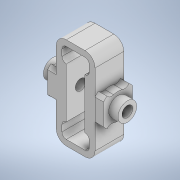
# Autodesk Inventor part: Součást3
Saved by Autodesk Inventor 2022 (Build 260153000, 153)
## iProperties
Created: 2022-04-03
Part Number: Součást3
Material: Všeobecné
Document SubType Name: Modeling
Designer: Šimon
Density: 1 g/cm^3
Appearance: Výchozí
Author: Šimon
Autodesk Inventor part; units mm, degrees
ref_plane "YZ Plane" through (0, 0, 0) normal (1, 0, 0) x (0, 1, 0)
ref_plane "XZ Plane" through (0, 0, 0) normal (0, 1, 0) x (-1, 0, 0)
ref_plane "XY Plane" through (0, 0, 0) normal (0, 0, 1) x (1, 0, 0)
sketch "Náčrt2" plane through (0, 0, 0) normal (0, 0, 1) x (1, 0, 0)
  line L0 (0, 0) -> (54, 0)
  line L1 (54, 0) -> (54, 128)
  line L2 (54, 128) -> (0, 128)
  line L3 (0, 128) -> (0, 0)
  line L4 (8, 120) -> (46, 120)
  line L5 (46, 120) -> (46, 99)
  line L6 (8, 99) -> (8, 120)
  line L7 (40, 99) -> (40, 29)
  line L8 (14, 29) -> (14, 99)
  line L9 (8, 29) -> (8, 8)
  line L10 (8, 8) -> (46, 8)
  line L11 (46, 8) -> (46, 29)
  line L12 (46, 99) -> (40, 99)
  line L13 (14, 99) -> (8, 99)
  line L14 (46, 29) -> (40, 29)
  line L15 (14, 29) -> (8, 29)
  point P0 (27, 120)
  point P1 (27, 128)
  dimension "d0" = 54
  dimension "d1" = 128
  dimension "d2" = 38
  dimension "d4" = 8
  dimension "d5" = 8
  dimension "d7" = 38
  dimension "d8" = 6
  dimension "d9" = 6
  constraints: 32 end point, 9 parallel, 4 horizontal, 4 perpendicular, 2 midpoint, 1 vertical alignment
  measures "d0" distance of L2.end L1.end
  measures "d1" distance of L0.end L1.end
  measures "d2" distance between parallel lines of L6 L5
  measures "d4" distance between parallel lines of L2 L4
  measures "d5" distance between parallel lines of L0 L10
  measures "d7" distance between parallel lines of L11 L9
  measures "d8" distance between parallel lines of L5 L7
  measures "d9" distance between parallel lines of L6 L8
extrude "Vysunutí1" add sketch "Náčrt2" along normal blind 40
fillet "Zaoblení1" radius 14 4 edges at (54, 128, 20) (0, 128, 20) (0, 0, 20) (54, 0, 20)
fillet "Zaoblení2" radius 6 8 edges at (8, 29, 20) (8, 99, 20) (46, 99, 20) (46, 120, 20) (8, 120, 20) (46, 8, 20) (8, 8, 20) (46, 29, 20)
sketch "Náčrt3" plane through (0, 0, 0) normal (1, 0, 0) x (0, 1, 0)
  circle A0 centre (64, 20) radius 13.0022
  line L0 (114, 0) -> (14, 0) projected
  line L1 (0, 0) -> (0, 40) projected
  dimension "d14" = 20
  dimension "d15" = 64
  constraints: 1 centre point
  measures "d14" distance from line of L0 A0.centre
  measures "d15" distance from line of L1 A0.centre
extrude "Vysunutí2" add sketch "Náčrt3" against normal blind 25
sketch "Náčrt4" plane through (54, 14, 0) normal (1, 0, 0) x (0, 0, -1)
  circle A0 centre (-20, 50) radius 13.0022 projected
  circle A1 centre (-20, 50) radius 13.0022
  point P0 (0, -14)
  constraints: 1 centre point, 1 coincident
extrude "Vysunutí3" add sketch "Náčrt4" along normal blind 25
sketch "Náčrt5" plane through (79, 64, 20) normal (1, 0, 0) x (0, 0, -1)
  circle A0 centre (0, 0) radius 7.5
  point P0 (20, -64)
  dimension "d20" = 15
  constraints: 1 centre point
  measures "d20" diameter of A0
extrude "Vysunutí4" cut sketch "Náčrt5" against normal through all
sketch "Náčrt6" plane through (0, 14, 0) normal (-1, 0, 0) x (0, 0, 1)
  circle A0 centre (20, 50) radius 7.5 projected
  line L0 (-4, 50) -> (52, 50)
  line L1 (0, 65) -> (0, 35)
  line L2 (40, 65) -> (40, 35)
  arc A1 (26.1564, 66.9145) -> (13.8436, 66.9145) centre (20, 50) ccw
  line L3 (20, 50) -> (8.6061, 81.3045) construction
  line L4 (20, 50) -> (31.3939, 81.3045) construction
  arc A2 (4.6393, 69.7243) -> (13.8436, 66.9145) centre (11.1075, 74.432) ccw
  arc A3 (26.1564, 66.9145) -> (35.3607, 69.7243) centre (28.8925, 74.432) ccw
  arc A4 (40, 65) -> (35.3607, 69.7243) centre (20, 50) ccw
  arc A5 (4.6393, 69.7243) -> (0, 65) centre (20, 50) ccw
  arc A6 (13.8436, 33.0855) -> (4.6393, 30.2757) centre (11.1075, 25.568) ccw
  arc A7 (13.8436, 33.0855) -> (26.1564, 33.0855) centre (20, 50) ccw
  arc A8 (35.3607, 30.2757) -> (26.1564, 33.0855) centre (28.8925, 25.568) ccw
  arc A9 (0, 35) -> (4.6393, 30.2757) centre (20, 50) ccw
  arc A10 (35.3607, 30.2757) -> (40, 35) centre (20, 50) ccw
  dimension "d27" = 36
  dimension "d28" = 40
  dimension "d29" = 8
  dimension "d30" = 25
  constraints: 20 point on circle, 10 centre point, 10 end point, 6 symmetric about line, 4 point on line, 1 coincident, 1 tangent, 3 other
  measures "d27" diameter of A1
  measures "d28" angle of L4 L3
  measures "d29" radius of A2
  measures "d30" radius of A5
extrude "Vysunutí5" add sketch "Náčrt6" along normal blind 12 contours L0 L2 A10 A8 A7 A6 A9 L1 A0 | A0 L0 L1 A5 A2 A1 A3 A4 L2
sketch "Náčrt7" plane through (54, 14, 0) normal (1, 0, 0) x (0, 0, -1)
  circle A0 centre (-20.0271, 50) radius 7.5
  line L0 (-44.0271, 50) -> (11.9729, 50)
  line L1 (-0.0271, 65) -> (-0.0271, 35)
  line L2 (-40.0271, 65) -> (-40.0271, 35)
  arc A1 (-13.8707, 66.9145) -> (-26.1834, 66.9145) centre (-20.0271, 50) ccw
  arc A2 (-0.0271, 65) -> (-4.6663, 69.7243) centre (-20.0271, 50) ccw
  arc A3 (-13.8707, 66.9145) -> (-4.6663, 69.7243) centre (-11.1345, 74.432) ccw
  arc A4 (-35.3878, 69.7243) -> (-40.0271, 65) centre (-20.0271, 50) ccw
  line L3 (-20.0271, 50) -> (-8.6332, 81.3045) construction
  line L4 (-20.0271, 50) -> (-31.421, 81.3045) construction
  arc A5 (-35.3878, 69.7243) -> (-26.1834, 66.9145) centre (-28.9196, 74.432) ccw
  arc A6 (-4.6663, 30.2757) -> (-0.0271, 35) centre (-20.0271, 50) ccw
  arc A7 (-4.6663, 30.2757) -> (-13.8707, 33.0855) centre (-11.1345, 25.568) ccw
  arc A8 (-26.1834, 33.0855) -> (-13.8707, 33.0855) centre (-20.0271, 50) ccw
  arc A9 (-26.1834, 33.0855) -> (-35.3878, 30.2757) centre (-28.9196, 25.568) ccw
  arc A10 (-40.0271, 35) -> (-35.3878, 30.2757) centre (-20.0271, 50) ccw
  point P0 (0, -14)
  dimension "d33" = 36
  dimension "d34" = 40
  dimension "d35" = 8
  dimension "d36" = 25
  constraints: 20 point on circle, 11 centre point, 10 end point, 6 symmetric about line, 4 point on line, 1 coincident, 1 tangent, 3 other
  measures "d33" diameter of A1
  measures "d34" angle of L3 L4
  measures "d35" radius of A5
  measures "d36" radius of A4
extrude "Vysunutí6" add sketch "Náčrt7" along normal blind 12 contours L0 L1 A6 A7 A8 A9 A10 L2 A0 | A0 L0 L2 A4 A5 A1 A3 A2 L1
